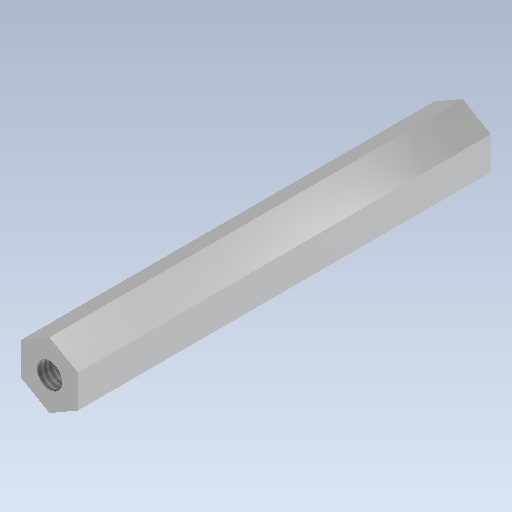
# Autodesk Inventor part: ASU-340
Saved by Autodesk Inventor 2020 (Build 240168000, 168)
## iProperties
Created: 2016-05-27
Part Number: ASU-340
Material: ステンレス鋼 AISI 304
Document SubType Name: Modeling
Designer: hiroaki
Density: 8 g/cm^3
Appearance: クローム - サテン
Mass: 7.92722 g
Surface Area: 9.07199 cm^2
Volume: 0.990902 cm^3
Author: hiroaki
Autodesk Inventor part; units mm, degrees
ref_plane "YZ Plane" through (0, 0, 0) normal (1, 0, 0) x (0, 1, 0)
ref_plane "XZ Plane" through (0, 0, 0) normal (0, 1, 0) x (-1, 0, 0)
ref_plane "XY Plane" through (0, 0, 0) normal (0, 0, 1) x (1, 0, 0)
sketch "スケッチ1" plane through (0, 0, 0) normal (0, 0, 1) x (1, 0, 0)
  line L0 (2.75, 1.5877) -> (2.75, -1.5877)
  line L1 (2.75, -1.5877) -> (0, -3.1754)
  line L2 (0, -3.1754) -> (-2.75, -1.5877)
  line L3 (-2.75, -1.5877) -> (-2.75, 1.5877)
  line L4 (-2.75, 1.5877) -> (0, 3.1754)
  line L5 (0, 3.1754) -> (2.75, 1.5877)
  point P0 (0, 0)
  point P1 (0, 0)
  dimension "d0" = 5.5
  constraints: 12 end point, 1 coincident, 1 vertical, 13 other
  measures "d0" distance between parallel lines of L0 L3
extrude "押し出し1" add sketch "スケッチ1" along normal blind 20
sketch "スケッチ2" plane through (0, 0, 20) normal (0, 0, 1) x (1, 0, 0)
  point P0 (0, 0)
  point P1 (0, 0)
  constraints: 1 coincident
hole "穴1" at (0, 0, 20) direction (0, 0, -1) diameter 2.459 depth 6 thread size "M3x0.5" class "6H" standard "ISO Metric profile"
mirror "ミラー1" about plane through (0, 0, 0) normal (0, 0, -1) of "押し出し1", "穴1"
